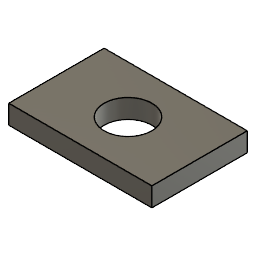
tr1 (Autodesk Fusion 360 design; units mm, degrees)
part number: 2026-08-20-00-00-46-151
Autodesk Fusion 360 part; units mm, degrees
sketch "Sketch1" plane through (0, 0, 0) normal (0, 1, 0) x (1, 0, 0)
  line L0 (75, 50) -> (-75, 50)
  line L1 (-75, 50) -> (-75, -50)
  line L2 (-75, -50) -> (75, -50)
  line L3 (75, -50) -> (75, 50)
  line L4 (75, 50) -> (-75, -50) construction
  line L5 (-75, 50) -> (75, -50) construction
  constraint horizontal L0
  constraint perpendicular L0 L1
  constraint parallel L0 L2
  constraint parallel L1 L3
  constraint coincident L4 origin
  constraint coincident L5 origin
extrude "Extrude1" add sketch "Sketch1" along normal blind 20
sketch "Sketch2" plane through (0, 20, 0) normal (0, 1, 0) x (-1, 0, 0)
  line L0 (-75, 50) -> (-75, -50)
  line L1 (-75, -50) -> (75, -50)
  line L2 (75, -50) -> (75, 50)
  line L3 (75, 50) -> (-75, 50)
  circle A0 centre (0, 0) radius 25
  constraint coincident A0.centre origin
extrude "Extrude2" cut sketch "Sketch2" against normal blind 20 contours A0
